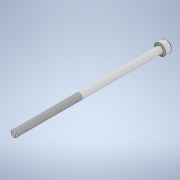
# Autodesk Inventor part: screw_4_90
Saved by Autodesk Inventor 2020 (Build 240168000, 168)
## iProperties
Created: 2020-08-18
Part Number: screw_4_90
Material: Generic
Document SubType Name: Modeling
Designer: psrobotics
Density: 1 g/cm^3
Appearance: Default
Author: psrobotics
Autodesk Inventor part; units mm, degrees
ref_plane "YZ Plane" through (0, 0, 0) normal (1, 0, 0) x (0, 1, 0)
ref_plane "XZ Plane" through (0, 0, 0) normal (0, 1, 0) x (-1, 0, 0)
ref_plane "XY Plane" through (0, 0, 0) normal (0, 0, 1) x (1, 0, 0)
sketch "Sketch1" plane through (0, 0, 0) normal (0, 1, 0) x (-1, 0, 0)
  line L0 (0, 0) -> (2, 0)
  line L1 (2, 0) -> (2, 90)
  line L2 (2, 90) -> (0, 90)
  line L3 (0, 90) -> (0, 0)
  line L4 (0, 0) -> (3.5, 0)
  line L5 (3.5, 0) -> (3.5, -4)
  line L6 (3.5, -4) -> (0, -4)
  line L7 (0, -4) -> (0, 0)
  dimension "d0" = 2
  dimension "d1" = 90
  dimension "d2" = 3.5
  dimension "d3" = 4
  constraints: 16 end point, 4 parallel, 2 horizontal, 2 perpendicular
  measures "d0" distance of L2.end L1.end
  measures "d1" distance of L1.end L0.end
  measures "d2" distance of L5.end L6.end
  measures "d3" distance of L4.end L5.end
revolve "Revolution1" add sketch "Sketch1" angle 360 about axis through (0, 0, 90) along (0, 0, -1)
chamfer "Chamfer1" distance 0.5 angle 45 2 edges at (2, 0, 90) (3.5, 0, -4)
thread "Thread1" size "M4x0.7" class "6g" standard "ANSI Metric M Profile" length 40
sketch "Sketch2" plane through (0, 0, -4) normal (0, 0, -1) x (-1, 0, 0)
  line L0 (0, 0) -> (1.5, 0)
  line L1 (0, 0) -> (0.75, 1.299)
  line L2 (0, 0) -> (-0.75, 1.299)
  line L3 (0, 0) -> (-1.5, 0)
  line L4 (0, 0) -> (-0.75, -1.299)
  line L5 (0, 0) -> (0.75, -1.299)
  line L6 (0.75, 1.299) -> (1.5, 0)
  line L7 (1.5, 0) -> (0.75, -1.299)
  circle A0 centre (0, 0) radius 1.5 projected
  line L8 (0.75, -1.299) -> (-0.75, -1.299)
  line L9 (-0.75, -1.299) -> (-1.5, 0)
  line L10 (-1.5, 0) -> (-0.75, 1.299)
  line L11 (-0.75, 1.299) -> (0.75, 1.299)
  dimension "d10" = 1.5
  dimension "d13" = 360
  constraints: 24 end point, 2 coincident, 1 horizontal, 1 parallel, 1 point on line, 19 other
  measures "d10" distance of L0.start L0.end
extrude "Extrusion1" cut sketch "Sketch2" against normal blind 2 contours L1 L6 L0 | L2 L11 L1 | L3 L10 L2 | L4 L9 L3 | L5 L8 L4 | L0 L7 L5
body "Solid1"
